Autodesk Inventor part; units mm, degrees
(part 2 of 2)
  spline S37 degree 3 poles (-24.7663, -45.875) (-24.7655, -45.8904) (-24.7641, -45.9208) (-24.7571, -45.9652) (-24.7471, -46.0075) (-24.7329, -46.0476) (-24.7153, -46.0857) (-24.6943, -46.1217) (-24.6693, -46.1555) (-24.641, -46.1868) (-24.6103, -46.2155) (-24.5771, -46.2402) (-24.5422, -46.2611) (-24.5058, -46.2786) (-24.4674, -46.2917) (-24.4273, -46.3015) (-24.3854, -46.3073) (-24.3569, -46.308) (-24.3423, -46.3083) knots 0 0 0 0 0.068791 0.135103 0.198979 0.261904 0.323495 0.385195 0.446969 0.509765 0.572251 0.633405 0.693251 0.752583 0.812579 0.873275 0.93555 1 1 1 1
  spline S38 degree 3 poles (-24.3423, -46.3083) (-24.3281, -46.308) (-24.3001, -46.3073) (-24.2592, -46.3017) (-24.2203, -46.2929) (-24.1834, -46.2805) (-24.1489, -46.2638) (-24.1164, -46.2439) (-24.0856, -46.2208) (-24.0579, -46.1935) (-24.0325, -46.1645) (-24.0105, -46.1335) (-23.9917, -46.1015) (-23.976, -46.0682) (-23.9645, -46.0333) (-23.9557, -45.9974) (-23.9508, -45.96) (-23.95, -45.9347) (-23.9496, -45.9218) knots 0 0 0 0 0.069475 0.136517 0.200789 0.26383 0.325735 0.387291 0.449509 0.512968 0.576275 0.63758 0.697903 0.757172 0.816599 0.876653 0.93729 1 1 1 1
  spline S39 degree 3 poles (-23.9496, -45.9218) (-23.9503, -45.9037) (-23.9515, -45.8678) (-23.9622, -45.8151) (-23.9788, -45.764) (-23.9989, -45.7229) (-24.0191, -45.6897) (-24.0374, -45.6624) (-24.0587, -45.633) (-24.0835, -45.6017) (-24.1111, -45.568) (-24.142, -45.5322) (-24.1762, -45.4945) (-24.2002, -45.4688) (-24.2127, -45.4554) knots 0 0 0 0 0.098702 0.195672 0.292422 0.391343 0.444462 0.504229 0.570352 0.642546 0.722288 0.807921 0.90047 1 1 1 1
  line L97 (-24.2127, -45.4554) -> (-24.5379, -45.1083)
  line L98 (-24.5379, -45.1083) -> (-23.933, -45.1083)
  line L99 (-23.933, -45.1083) -> (-23.933, -44.975)
  line L100 (-23.933, -44.975) -> (-24.8163, -44.975)
  line L101 (-24.8163, -44.975) -> (-24.3121, -45.513)
  spline S40 degree 3 poles (-24.3121, -45.513) (-24.2999, -45.5258) (-24.2763, -45.5504) (-24.2429, -45.5863) (-24.213, -45.6197) (-24.1862, -45.6504) (-24.1633, -45.6788) (-24.1429, -45.7041) (-24.1266, -45.7275) (-24.1088, -45.7545) (-24.0917, -45.7875) (-24.0769, -45.8278) (-24.0679, -45.8693) (-24.0669, -45.8973) (-24.0663, -45.9114) knots 0 0 0 0 0.110803 0.212829 0.306101 0.390647 0.466924 0.534481 0.593587 0.644557 0.7362 0.825024 0.911986 1 1 1 1
  line L102 (-23.5563, -45.625) -> (-23.423, -46.275)
  line L103 (-23.423, -46.275) -> (-22.8896, -46.275)
  line L104 (-22.8896, -46.275) -> (-22.8896, -46.1416)
  line L105 (-22.8896, -46.1416) -> (-23.3318, -46.1416)
  line L106 (-23.3318, -46.1416) -> (-23.4019, -45.7997)
  spline S41 degree 3 poles (-23.4019, -45.7997) (-23.3881, -45.8035) (-23.3615, -45.8109) (-23.3221, -45.819) (-23.2847, -45.824) (-23.2605, -45.8246) (-23.2488, -45.825) knots 0 0 0 0 0.275068 0.532901 0.773973 1 1 1 1
  spline S42 degree 3 poles (-23.2488, -45.825) (-23.2342, -45.8247) (-23.2057, -45.824) (-23.1639, -45.8181) (-23.1241, -45.8088) (-23.0862, -45.7957) (-23.0502, -45.779) (-23.0165, -45.7582) (-22.9845, -45.7339) (-22.9548, -45.7059) (-22.9278, -45.6751) (-22.9041, -45.642) (-22.884, -45.6068) (-22.8679, -45.5694) (-22.8549, -45.5301) (-22.8463, -45.4884) (-22.8406, -45.4447) (-22.84, -45.4149) (-22.8396, -45.3997) knots 0 0 0 0 0.065808 0.129394 0.190894 0.251281 0.310815 0.370371 0.430768 0.492881 0.555104 0.616067 0.677256 0.73826 0.800762 0.864778 0.931045 1 1 1 1
  spline S43 degree 3 poles (-22.8396, -45.3997) (-22.8399, -45.3891) (-22.8404, -45.3681) (-22.8429, -45.3368) (-22.8477, -45.3062) (-22.8541, -45.2763) (-22.8625, -45.2471) (-22.8726, -45.2185) (-22.885, -45.1907) (-22.8986, -45.1635) (-22.914, -45.1374) (-22.931, -45.113) (-22.9489, -45.0899) (-22.9683, -45.0685) (-22.9891, -45.0487) (-23.0113, -45.0305) (-23.0346, -45.0136) (-23.0593, -44.9987) (-23.085, -44.985) (-23.112, -44.9737) (-23.1397, -44.9636) (-23.1684, -44.9556) (-23.1981, -44.9493) (-23.229, -44.945) (-23.2607, -44.9419) (-23.2822, -44.9417) (-23.293, -44.9416) knots 0 0 0 0 0.044014 0.087434 0.130118 0.172554 0.214555 0.256298 0.298438 0.340849 0.382715 0.423924 0.464246 0.504074 0.543862 0.583567 0.623094 0.663229 0.703551 0.743938 0.784541 0.82575 0.867757 0.910745 0.954914 1 1 1 1
  spline S44 degree 3 poles (-23.293, -44.9416) (-23.306, -44.9419) (-23.3315, -44.9424) (-23.3688, -44.9477) (-23.4047, -44.9552) (-23.4389, -44.9666) (-23.4718, -44.9809) (-23.5028, -44.9989) (-23.5327, -45.0193) (-23.5604, -45.0434) (-23.5861, -45.0698) (-23.609, -45.0983) (-23.6295, -45.1287) (-23.6472, -45.161) (-23.6622, -45.1951) (-23.674, -45.2312) (-23.6836, -45.269) (-23.6876, -45.2951) (-23.6896, -45.3083) knots 0 0 0 0 0.065421 0.128708 0.190236 0.250724 0.310637 0.370766 0.431615 0.493523 0.555883 0.617342 0.678668 0.740711 0.802985 0.866803 0.932347 1 1 1 1
  line L107 (-23.6896, -45.3083) -> (-23.573, -45.3083)
  spline S45 degree 3 poles (-23.573, -45.3083) (-23.5701, -45.2959) (-23.5646, -45.2721) (-23.5525, -45.2386) (-23.5377, -45.2088) (-23.5201, -45.1822) (-23.4991, -45.159) (-23.4751, -45.1383) (-23.4482, -45.1197) (-23.4184, -45.1042) (-23.3869, -45.0909) (-23.3539, -45.0821) (-23.3203, -45.0759) (-23.2977, -45.0753) (-23.2863, -45.075) knots 0 0 0 0 0.094687 0.181994 0.264377 0.34218 0.418618 0.496509 0.577369 0.661511 0.746733 0.831258 0.915206 1 1 1 1
  spline S46 degree 3 poles (-23.2863, -45.075) (-23.2751, -45.0753) (-23.2532, -45.0759) (-23.221, -45.0805) (-23.1898, -45.0876) (-23.1601, -45.0983) (-23.1313, -45.1112) (-23.1041, -45.1278) (-23.0778, -45.1469) (-23.0531, -45.1688) (-23.0305, -45.1929) (-23.0106, -45.2188) (-22.9939, -45.2463) (-22.9799, -45.2751) (-22.9693, -45.3054) (-22.9617, -45.3372) (-22.9572, -45.3704) (-22.9566, -45.3931) (-22.9563, -45.4047) knots 0 0 0 0 0.064207 0.126425 0.18768 0.248216 0.308305 0.369661 0.431699 0.495947 0.559758 0.622295 0.683911 0.745092 0.80674 0.869087 0.93329 1 1 1 1
  spline S47 degree 3 poles (-22.9563, -45.4047) (-22.9566, -45.4151) (-22.957, -45.4355) (-22.9609, -45.4654) (-22.9677, -45.4936) (-22.9772, -45.5204) (-22.9892, -45.5457) (-23.0038, -45.5697) (-23.0214, -45.5918) (-23.0415, -45.6123) (-23.0635, -45.6312) (-23.0878, -45.6473) (-23.1139, -45.6608) (-23.1415, -45.6725) (-23.1712, -45.6809) (-23.2024, -45.6872) (-23.2356, -45.6909) (-23.2582, -45.6914) (-23.2698, -45.6916) knots 0 0 0 0 0.065351 0.127916 0.18836 0.247216 0.30563 0.36377 0.422661 0.482687 0.5433 0.604118 0.664965 0.727413 0.791468 0.858055 0.927037 1 1 1 1
  spline S48 degree 3 poles (-23.2698, -45.6916) (-23.2799, -45.6914) (-23.3007, -45.691) (-23.3326, -45.6877) (-23.3662, -45.6824) (-23.4012, -45.6751) (-23.4378, -45.6656) (-23.476, -45.6542) (-23.5158, -45.6406) (-23.5425, -45.6303) (-23.5563, -45.625) knots 0 0 0 0 0.102203 0.211023 0.3251 0.446502 0.573788 0.708901 0.850358 1 1 1 1
  line L108 (-20.1096, -44.975) -> (-19.493, -46.275)
  line L109 (-19.493, -46.275) -> (-19.4763, -46.275)
  line L110 (-19.4763, -46.275) -> (-18.8763, -44.975)
  line L111 (-18.8763, -44.975) -> (-19.0031, -44.975)
  line L112 (-19.0031, -44.975) -> (-19.1953, -45.3916)
  line L113 (-19.1953, -45.3916) -> (-19.7846, -45.3916)
  line L114 (-19.7846, -45.3916) -> (-19.9823, -44.975)
  line L115 (-19.9823, -44.975) -> (-20.1096, -44.975)
  spline S49 degree 3 poles (-18.5996, -45.6325) (-18.5991, -45.6559) (-18.5979, -45.7019) (-18.5883, -45.7694) (-18.5727, -45.8341) (-18.5507, -45.8958) (-18.5227, -45.9549) (-18.4882, -46.011) (-18.4474, -46.0643) (-18.4008, -46.1141) (-18.3497, -46.1596) (-18.295, -46.1996) (-18.2368, -46.2329) (-18.1757, -46.2608) (-18.1112, -46.2822) (-18.0436, -46.2972) (-17.9729, -46.3065) (-17.9247, -46.3077) (-17.9002, -46.3083) knots 0 0 0 0 0.064558 0.127014 0.187955 0.248014 0.307748 0.368235 0.42947 0.492743 0.556258 0.618217 0.679655 0.741246 0.803415 0.866815 0.932328 1 1 1 1
  spline S50 degree 3 poles (-17.9002, -46.3083) (-17.8852, -46.3081) (-17.8557, -46.3078) (-17.8119, -46.3043) (-17.7693, -46.2985) (-17.7279, -46.2907) (-17.6874, -46.281) (-17.6481, -46.2683) (-17.6098, -46.2538) (-17.5727, -46.2371) (-17.5371, -46.2183) (-17.5029, -46.1978) (-17.4704, -46.1754) (-17.4394, -46.1513) (-17.4104, -46.1252) (-17.3825, -46.0976) (-17.3568, -46.0679) (-17.3409, -46.0469) (-17.333, -46.0364) knots 0 0 0 0 0.068548 0.135683 0.201215 0.265682 0.329267 0.392395 0.45507 0.517127 0.57879 0.63974 0.700192 0.759806 0.819628 0.879355 0.939512 1 1 1 1
  line L116 (-17.333, -46.0364) -> (-17.4351, -45.9583)
  spline S51 degree 3 poles (-17.4351, -45.9583) (-17.4423, -45.967) (-17.4568, -45.9842) (-17.4801, -46.0084) (-17.5043, -46.0311) (-17.5296, -46.0524) (-17.5562, -46.0715) (-17.5836, -46.0894) (-17.6123, -46.1055) (-17.652, -46.125) (-17.7038, -46.1453) (-17.7691, -46.1623) (-17.8373, -46.1732) (-17.8838, -46.1744) (-17.9075, -46.175) knots 0 0 0 0 0.063163 0.125475 0.187121 0.248294 0.309295 0.36985 0.430973 0.492456 0.616148 0.740844 0.868183 1 1 1 1
  spline S52 degree 3 poles (-17.9075, -46.175) (-17.9205, -46.1748) (-17.9464, -46.1745) (-17.9849, -46.1706) (-18.0227, -46.165) (-18.0597, -46.1568) (-18.096, -46.1464) (-18.1317, -46.134) (-18.1663, -46.1187) (-18.2003, -46.1017) (-18.2329, -46.0825) (-18.2638, -46.0616) (-18.2928, -46.0392) (-18.3199, -46.0151) (-18.3452, -45.9897) (-18.3685, -45.9624) (-18.3898, -45.9335) (-18.4094, -45.9033) (-18.4269, -45.8719) (-18.4416, -45.8392) (-18.4546, -45.8057) (-18.4649, -45.7711) (-18.473, -45.7356) (-18.4786, -45.6991) (-18.4825, -45.6618) (-18.4828, -45.6364) (-18.483, -45.6237) knots 0 0 0 0 0.043955 0.087502 0.130463 0.172752 0.215403 0.25765 0.300153 0.343121 0.385925 0.427686 0.468818 0.509492 0.549883 0.58998 0.630405 0.670869 0.711384 0.751627 0.791776 0.832459 0.873319 0.914543 0.956924 1 1 1 1
  spline S53 degree 3 poles (-18.483, -45.6237) (-18.4825, -45.6044) (-18.4816, -45.5667) (-18.4734, -45.5115) (-18.461, -45.4585) (-18.4423, -45.4082) (-18.4193, -45.36) (-18.3902, -45.3146) (-18.3566, -45.2714) (-18.3179, -45.2313) (-18.2754, -45.1947) (-18.2298, -45.1625) (-18.1812, -45.1356) (-18.1302, -45.1133) (-18.0763, -45.0961) (-18.0197, -45.084) (-17.9605, -45.0761) (-17.92, -45.0753) (-17.8994, -45.075) knots 0 0 0 0 0.064323 0.12629 0.186726 0.246146 0.305576 0.365429 0.426326 0.48884 0.551725 0.613919 0.675484 0.737334 0.800229 0.864502 0.931041 1 1 1 1
  spline S54 degree 3 poles (-17.8994, -45.075) (-17.8767, -45.0756) (-17.832, -45.0768) (-17.7665, -45.0873) (-17.7038, -45.1042) (-17.6439, -45.128) (-17.5869, -45.1588) (-17.5328, -45.1962) (-17.4816, -45.2405) (-17.4508, -45.2744) (-17.4351, -45.2916) knots 0 0 0 0 0.128515 0.252949 0.374755 0.49594 0.617181 0.740909 0.867811 1 1 1 1
  line L117 (-17.4351, -45.2916) -> (-17.333, -45.2143)
  spline S55 degree 3 poles (-17.333, -45.2143) (-17.3412, -45.2037) (-17.3576, -45.1825) (-17.3841, -45.1527) (-17.4121, -45.1247) (-17.4417, -45.0986) (-17.4725, -45.0741) (-17.5053, -45.0517) (-17.5394, -45.0311) (-17.5748, -45.0123) (-17.6115, -44.9956) (-17.6494, -44.9814) (-17.6883, -44.9691) (-17.7283, -44.9589) (-17.7694, -44.951) (-17.8115, -44.9457) (-17.8547, -44.9421) (-17.8838, -44.9418) (-17.8986, -44.9416) knots 0 0 0 0 0.061674 0.123053 0.183475 0.243727 0.304279 0.364863 0.425946 0.487391 0.54922 0.611144 0.673529 0.736961 0.800785 0.866013 0.932101 1 1 1 1
  spline S56 degree 3 poles (-17.8986, -44.9416) (-17.9126, -44.9417) (-17.9402, -44.9419) (-17.981, -44.945) (-18.0208, -44.9493) (-18.0593, -44.9557) (-18.0969, -44.9633) (-18.1331, -44.9734) (-18.1684, -44.9847) (-18.2026, -44.9981) (-18.2356, -45.0131) (-18.2675, -45.0301) (-18.2982, -45.0489) (-18.328, -45.0692) (-18.3565, -45.0914) (-18.3838, -45.1155) (-18.4102, -45.1411) (-18.4266, -45.1597) (-18.4348, -45.169) knots 0 0 0 0 0.069663 0.13775 0.203917 0.26878 0.332414 0.394754 0.45618 0.516996 0.577396 0.637198 0.696999 0.756756 0.816554 0.876948 0.938132 1 1 1 1
  spline S57 degree 3 poles (-18.4348, -45.169) (-18.448, -45.1851) (-18.4741, -45.2173) (-18.5076, -45.2694) (-18.5363, -45.3238) (-18.5594, -45.3808) (-18.5775, -45.4402) (-18.5901, -45.5022) (-18.5982, -45.5665) (-18.5992, -45.6103) (-18.5996, -45.6325) knots 0 0 0 0 0.124329 0.247156 0.36878 0.490734 0.613614 0.738958 0.867311 1 1 1 1
  line L118 (-15.527, -46.225) -> (-15.7398, -46.225)
  line L119 (-15.9273, -45.125) -> (-15.527, -46.225)
  line L120 (-15.4273, -45.125) -> (-15.9273, -45.125)
  line L121 (-15.027, -46.225) -> (-15.4273, -45.125)
  line L122 (-14.8141, -46.225) -> (-15.027, -46.225)
  line L123 (-15.2145, -45.125) -> (-14.8141, -46.225)
  line L124 (-15.0145, -45.125) -> (-15.2145, -45.125)
  line L125 (-15.0873, -44.925) -> (-15.0145, -45.125)
  line L126 (-16.213, -44.925) -> (-15.0873, -44.925)
  line L127 (-15.7398, -46.225) -> (-16.213, -44.925)
  line L128 (-20.903, -44.975) -> (-20.9196, -44.975)
  line L129 (-20.9196, -44.975) -> (-21.4696, -46.275)
  line L130 (-21.4696, -46.275) -> (-21.3446, -46.275)
  line L131 (-21.3446, -46.275) -> (-20.9113, -45.2505)
  line L132 (-20.9113, -45.2505) -> (-20.478, -46.275)
  line L133 (-20.478, -46.275) -> (-20.353, -46.275)
  line L134 (-20.353, -46.275) -> (-20.903, -44.975)
  spline S58 degree 3 poles (-21.713, -45.6244) (-21.7132, -45.6046) (-21.7137, -45.5658) (-21.7161, -45.5092) (-21.7209, -45.4557) (-21.727, -45.4052) (-21.7353, -45.3581) (-21.7456, -45.3139) (-21.7569, -45.2727) (-21.771, -45.2348) (-21.7864, -45.1995) (-21.8031, -45.1666) (-21.821, -45.1357) (-21.8406, -45.1071) (-21.8614, -45.0806) (-21.8839, -45.0566) (-21.9076, -45.0346) (-21.9326, -45.0151) (-21.9588, -44.998) (-21.9855, -44.9826) (-22.0133, -44.9703) (-22.0415, -44.9597) (-22.0705, -44.9516) (-22.1003, -44.946) (-22.1308, -44.9421) (-22.1513, -44.9418) (-22.1617, -44.9416) knots 0 0 0 0 0.065063 0.126773 0.185516 0.240765 0.29298 0.34225 0.388919 0.432776 0.474628 0.514775 0.553606 0.591426 0.628028 0.663804 0.698984 0.733591 0.767628 0.801208 0.834264 0.866981 0.89972 0.932702 0.966176 1 1 1 1
  spline S59 degree 3 poles (-22.1617, -44.9416) (-22.1719, -44.9418) (-22.1921, -44.9421) (-22.2221, -44.9457) (-22.2512, -44.9514) (-22.2795, -44.9593) (-22.3073, -44.9691) (-22.334, -44.9817) (-22.3601, -44.9963) (-22.3855, -45.013) (-22.4097, -45.032) (-22.4327, -45.0531) (-22.4541, -45.0768) (-22.4741, -45.1026) (-22.493, -45.1303) (-22.5104, -45.1604) (-22.5265, -45.1926) (-22.5412, -45.2273) (-22.5543, -45.2649) (-22.5658, -45.3058) (-22.5749, -45.3504) (-22.5827, -45.3983) (-22.589, -45.4499) (-22.5933, -45.5049) (-22.596, -45.5636) (-22.5962, -45.6038) (-22.5963, -45.6244) knots 0 0 0 0 0.033787 0.066622 0.099285 0.131361 0.163585 0.196104 0.228902 0.262158 0.295991 0.330218 0.36506 0.400951 0.43762 0.475708 0.515381 0.556414 0.599765 0.646424 0.696431 0.749782 0.806573 0.867436 0.931887 1 1 1 1
  spline S60 degree 3 poles (-22.5963, -45.6244) (-22.5962, -45.6453) (-22.5959, -45.6858) (-22.5933, -45.7447) (-22.5889, -45.8001) (-22.5829, -45.8517) (-22.5757, -45.8998) (-22.5659, -45.9441) (-22.5548, -45.9848) (-22.542, -46.0221) (-22.5275, -46.0565) (-22.5118, -46.0886) (-22.4941, -46.1184) (-22.4755, -46.1463) (-22.4553, -46.1719) (-22.434, -46.1955) (-22.4109, -46.2166) (-22.3866, -46.2359) (-22.3609, -46.2528) (-22.3347, -46.2677) (-22.3077, -46.2804) (-22.2798, -46.2903) (-22.2513, -46.2986) (-22.2221, -46.3042) (-22.1921, -46.3078) (-22.1719, -46.3081) (-22.1617, -46.3083) knots 0 0 0 0 0.068595 0.133246 0.194313 0.251279 0.304513 0.354235 0.400481 0.443411 0.484015 0.523252 0.561042 0.5979 0.633518 0.668314 0.702496 0.736685 0.770293 0.803437 0.835913 0.86846 0.900847 0.933467 0.966258 1 1 1 1
  spline S61 degree 3 poles (-22.1617, -46.3083) (-22.1513, -46.3081) (-22.1308, -46.3078) (-22.1004, -46.3043) (-22.0707, -46.2985) (-22.0418, -46.2904) (-22.0135, -46.2803) (-21.9861, -46.2676) (-21.9593, -46.2529) (-21.9335, -46.2356) (-21.9085, -46.2163) (-21.885, -46.1945) (-21.8628, -46.1703) (-21.8418, -46.1442) (-21.8224, -46.1155) (-21.804, -46.0847) (-21.7875, -46.0514) (-21.7717, -46.016) (-21.7579, -45.9777) (-21.7456, -45.9365) (-21.7356, -45.8921) (-21.7273, -45.8447) (-21.7209, -45.794) (-21.7162, -45.7402) (-21.7137, -45.6833) (-21.7132, -45.6444) (-21.713, -45.6244) knots 0 0 0 0 0.033788 0.067194 0.099862 0.132567 0.165151 0.197913 0.231319 0.265083 0.299255 0.334399 0.369943 0.406284 0.444064 0.482998 0.523354 0.565537 0.609613 0.656391 0.705885 0.758325 0.813832 0.872795 0.934722 1 1 1 1
  line L135 (-27.863, -45.625) -> (-27.7296, -46.275)
  line L136 (-27.7296, -46.275) -> (-27.1963, -46.275)
  line L137 (-27.1963, -46.275) -> (-27.1963, -46.1416)
  line L138 (-27.1963, -46.1416) -> (-27.6385, -46.1416)
  line L139 (-27.6385, -46.1416) -> (-27.7085, -45.7997)
  spline S62 degree 3 poles (-27.7085, -45.7997) (-27.6948, -45.8035) (-27.6681, -45.8109) (-27.6288, -45.819) (-27.5914, -45.824) (-27.5672, -45.8246) (-27.5554, -45.825) knots 0 0 0 0 0.275068 0.532901 0.773973 1 1 1 1
  spline S63 degree 3 poles (-27.5554, -45.825) (-27.5409, -45.8247) (-27.5124, -45.824) (-27.4706, -45.8181) (-27.4307, -45.8088) (-27.3928, -45.7957) (-27.3569, -45.779) (-27.3231, -45.7582) (-27.2911, -45.7339) (-27.2614, -45.7059) (-27.2345, -45.6751) (-27.2108, -45.642) (-27.1907, -45.6068) (-27.1745, -45.5694) (-27.1616, -45.5301) (-27.153, -45.4884) (-27.1473, -45.4447) (-27.1466, -45.4149) (-27.1463, -45.3997) knots 0 0 0 0 0.065808 0.129394 0.190894 0.251281 0.310815 0.370371 0.430768 0.492881 0.555104 0.616067 0.677256 0.73826 0.800762 0.864778 0.931045 1 1 1 1
  spline S64 degree 3 poles (-27.1463, -45.3997) (-27.1466, -45.3891) (-27.147, -45.3681) (-27.1495, -45.3368) (-27.1543, -45.3062) (-27.1608, -45.2763) (-27.1692, -45.2471) (-27.1793, -45.2185) (-27.1917, -45.1907) (-27.2053, -45.1635) (-27.2206, -45.1374) (-27.2376, -45.113) (-27.2556, -45.0899) (-27.2749, -45.0685) (-27.2958, -45.0487) (-27.318, -45.0305) (-27.3413, -45.0136) (-27.366, -44.9987) (-27.3917, -44.985) (-27.4187, -44.9737) (-27.4463, -44.9636) (-27.4751, -44.9556) (-27.5048, -44.9493) (-27.5356, -44.945) (-27.5673, -44.9419) (-27.5888, -44.9417) (-27.5997, -44.9416) knots 0 0 0 0 0.044014 0.087434 0.130118 0.172554 0.214555 0.256298 0.298438 0.340849 0.382715 0.423924 0.464246 0.504074 0.543862 0.583567 0.623094 0.663229 0.703551 0.743938 0.784541 0.82575 0.867757 0.910745 0.954914 1 1 1 1
  spline S65 degree 3 poles (-27.5997, -44.9416) (-27.6126, -44.9419) (-27.6381, -44.9424) (-27.6755, -44.9477) (-27.7114, -44.9552) (-27.7456, -44.9666) (-27.7784, -44.9809) (-27.8094, -44.9989) (-27.8394, -45.0193) (-27.867, -45.0434) (-27.8927, -45.0698) (-27.9157, -45.0983) (-27.9362, -45.1287) (-27.9538, -45.161) (-27.9689, -45.1951) (-27.9807, -45.2312) (-27.9902, -45.269) (-27.9943, -45.2951) (-27.9963, -45.3083) knots 0 0 0 0 0.065421 0.128708 0.190236 0.250724 0.310637 0.370766 0.431615 0.493523 0.555883 0.617342 0.678668 0.740711 0.802985 0.866803 0.932347 1 1 1 1
  line L140 (-27.9963, -45.3083) -> (-27.8796, -45.3083)
  spline S66 degree 3 poles (-27.8796, -45.3083) (-27.8768, -45.2959) (-27.8713, -45.2721) (-27.8591, -45.2386) (-27.8443, -45.2088) (-27.8267, -45.1822) (-27.8057, -45.159) (-27.7818, -45.1383) (-27.7549, -45.1197) (-27.725, -45.1042) (-27.6935, -45.0909) (-27.6606, -45.0821) (-27.627, -45.0759) (-27.6043, -45.0753) (-27.5929, -45.075) knots 0 0 0 0 0.094687 0.181994 0.264377 0.34218 0.418618 0.496509 0.577369 0.661511 0.746733 0.831258 0.915206 1 1 1 1
  spline S67 degree 3 poles (-27.5929, -45.075) (-27.5818, -45.0753) (-27.5599, -45.0759) (-27.5276, -45.0805) (-27.4965, -45.0876) (-27.4668, -45.0983) (-27.438, -45.1112) (-27.4108, -45.1278) (-27.3845, -45.1469) (-27.3598, -45.1688) (-27.3372, -45.1929) (-27.3172, -45.2188) (-27.3006, -45.2463) (-27.2866, -45.2751) (-27.276, -45.3054) (-27.2684, -45.3372) (-27.2639, -45.3704) (-27.2633, -45.3931) (-27.263, -45.4047) knots 0 0 0 0 0.064207 0.126425 0.18768 0.248216 0.308305 0.369661 0.431699 0.495947 0.559758 0.622295 0.683911 0.745092 0.80674 0.869087 0.93329 1 1 1 1
  spline S68 degree 3 poles (-27.263, -45.4047) (-27.2632, -45.4151) (-27.2637, -45.4355) (-27.2676, -45.4654) (-27.2744, -45.4936) (-27.2839, -45.5204) (-27.2958, -45.5457) (-27.3105, -45.5697) (-27.3281, -45.5918) (-27.3482, -45.6123) (-27.3702, -45.6312) (-27.3945, -45.6473) (-27.4206, -45.6608) (-27.4482, -45.6725) (-27.4779, -45.6809) (-27.5091, -45.6872) (-27.5422, -45.6909) (-27.5649, -45.6914) (-27.5765, -45.6916) knots 0 0 0 0 0.065351 0.127916 0.18836 0.247216 0.30563 0.36377 0.422661 0.482687 0.5433 0.604118 0.664965 0.727413 0.791468 0.858055 0.927037 1 1 1 1
  spline S69 degree 3 poles (-27.5765, -45.6916) (-27.5866, -45.6914) (-27.6074, -45.691) (-27.6393, -45.6877) (-27.6728, -45.6824) (-27.7079, -45.6751) (-27.7445, -45.6656) (-27.7827, -45.6542) (-27.8224, -45.6406) (-27.8492, -45.6303) (-27.863, -45.625) knots 0 0 0 0 0.102203 0.211023 0.3251 0.446502 0.573788 0.708901 0.850358 1 1 1 1
  constraints: 282 end point, 138 symmetric about line, 60 point on circle, 36 horizontal, 34 centre point, 1 horizontal alignment, 162 other
extrude "Выдавливание28" cut sketch "Эскиз31" against normal blind 56.25 contours A15 | A16 | A33 | A34
